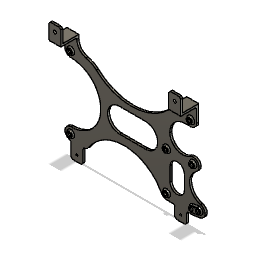
board-mounts (Autodesk Fusion 360 design; units mm, degrees)
Autodesk Fusion 360 part; units mm, degrees
sketch "test-screw-post" plane through (0, 0, 0) normal (0, 1, 0) x (1, 0, 0)
  line L0 (0, 0) -> (10, 0)
  line L1 (10, 0) -> (10, 10)
  line L2 (10, 10) -> (0, 10)
  line L3 (0, 10) -> (0, 0)
  circle A0 centre (5, 5) radius 1.55
  circle A1 centre (5, 5) radius 3.25
  dimension "d1" = 3.1
  dimension "d2" = 6.5
  dimension "d12" = 10
  constraint horizontal L0
  constraint vertical L1
  constraint horizontal L2
  constraint vertical L3
  constraint coincident L0.start L3.end
  constraint concentric A0 A1
  constraint equal L0 L1
  constraint collinear L0.end L2.end A0.centre
  constraint collinear L0.start L1.end A0.centre
  measures "d1" diameter of A0
  measures "d2" diameter of A1
  measures "d12" distance of L0.start L0.end
extrude "test-screw-post base" add sketch "test-screw-post" along normal blind 2.5 contours L0 L1 L2 L3 makes body 1
extrude "test-screw-post post" add sketch "test-screw-post" along normal blind 5 contours A1 bodies 1
fillet "test-screw-post post filet" radius 1.5 1 edges at (1.9699, 2.5, -6.1753) on bodies 1
chamfer "test-screw-post post hole chamfer" distance 0.75 angle 45 1 edges at (3.5549, 5, -5.5605) on bodies 1
sketch "mosfet-mount" plane through (0, 0, 0) normal (0, 0, 1) x (1, 0, 0)
  line L0 (31.2098, -47.0147) -> (36.1264, -47.3213)
  circle A0 centre (31.2098, -38.8279) radius 3.25
  arc A1 (27.187, -6.2985) -> (38.2098, -17.3213) centre (38.2098, -6.2985) ccw
  circle A2 centre (31.2098, -38.8279) radius 1.55
  arc A3 (23.3796, -41.2179) -> (31.2098, -47.0147) centre (31.2098, -38.8279) ccw
  arc A4 (23.3796, -41.2179) -> (1.2098, -24.8051) centre (1.2098, -47.9846) ccw
  line L1 (13.5336, -24.8051) -> (1.2098, -24.8051)
  line L2 (-11.1141, -24.8051) -> (1.2098, -24.8051)
  line L3 (1.2098, -24.8051) -> (1.2098, -17.3051)
  arc A5 (1.2098, -24.8051) -> (-20.9601, -41.2179) centre (1.2098, -47.9846) ccw
  circle A6 centre (-28.7902, -38.8279) radius 3.25
  circle A7 centre (-28.7902, -38.8279) radius 1.55
  line L4 (-35.7902, -47.0147) -> (-35.7902, -32.0147)
  arc A8 (19.687, 0.7275) -> (1.2098, 19.2047) centre (1.2098, 0.7275) ccw
  line L5 (27.187, 7.8914) -> (27.187, 0.7275)
  arc A9 (38.2098, 18.9143) -> (27.187, 7.8914) centre (38.2098, 7.8914) ccw
  arc A10 (1.2098, 26.7047) -> (23.3796, 43.1174) centre (1.2098, 49.8842) ccw
  line L6 (1.2098, 26.7047) -> (1.2098, 19.2047)
  arc A11 (1.2098, 19.2047) -> (-17.2674, 0.7275) centre (1.2098, 0.7275) ccw
  arc A12 (-20.9601, 43.1174) -> (1.2098, 26.7047) centre (1.2098, 49.8842) ccw
  line L7 (-11.1141, 26.7047) -> (1.2098, 26.7047)
  circle A13 centre (-28.7902, 40.7275) radius 3.25
  circle A14 centre (-28.7902, 40.7275) radius 1.55
  line L8 (-35.7902, 48.9143) -> (-35.7902, 33.9143)
  line L9 (-28.7902, 48.9143) -> (-35.7902, 48.9143)
  arc A15 (-20.9601, 43.1174) -> (-28.7902, 48.9143) centre (-28.7902, 40.7275) ccw
  circle A16 centre (31.2098, 40.7275) radius 3.25
  circle A17 centre (31.2098, 40.7275) radius 1.55
  line L10 (31.2098, 48.9143) -> (40.7098, 48.9143)
  line L11 (38.2098, 48.9143) -> (38.2098, 18.9143)
  line L12 (40.7098, 48.9143) -> (40.7098, 18.9143)
  arc A18 (31.2098, 48.9143) -> (23.3796, 43.1174) centre (31.2098, 40.7275) ccw
  arc A19 (-24.7674, 22.7238) -> (-35.7902, 33.9143) centre (-35.9591, 22.7238) ccw
  arc A20 (-35.7902, -32.0147) -> (-24.7674, -20.8242) centre (-35.9591, -20.8242) ccw
  arc A21 (-17.2674, 1.1721) -> (1.2098, -17.3051) centre (1.2098, 1.1721) ccw
  line L13 (27.187, -6.2985) -> (27.187, 1.1721)
  arc A22 (-28.7902, -47.0147) -> (-20.9601, -41.2179) centre (-28.7902, -38.8279) ccw
  line L14 (-28.7902, -47.0147) -> (-35.7902, -47.0147)
  line L15 (-8.7902, 0.9498) -> (10.2098, 0.9498)
  line L16 (11.2098, 0.9498) -> (-7.7902, 0.9498)
  line L17 (1.2098, 7) -> (1.2098, -7.7588)
  line L18 (-24.7674, 22.7238) -> (-24.7674, 0.7275)
  arc A23 (1.2098, -17.3051) -> (19.687, 1.1721) centre (1.2098, 1.1721) ccw
  line L19 (27.187, 1.1721) -> (19.687, 1.1721)
  line L20 (27.187, 0.7275) -> (19.687, 0.7275)
  line L21 (-24.7674, 1.1721) -> (-17.2674, 1.1721)
  line L22 (-24.7674, 0.7275) -> (-17.2674, 0.7275)
  line L23 (-24.7674, -20.8242) -> (-24.7674, 1.1721)
  line L24 (40.4687, -47.3213) -> (36.1264, -47.3213)
  line L25 (38.2098, -17.3213) -> (38.2098, -47.3213)
  line L26 (40.4687, -17.3213) -> (40.4687, -47.3213)
  line L27 (-35.7902, 48.9143) -> (-43.7902, 48.9143)
  line L28 (-45.7902, 46.9143) -> (-45.7902, 35.9143)
  line L29 (-43.7902, 33.9143) -> (-35.7902, 33.9143)
  line L30 (-35.7902, 33.9143) -> (-35.7902, 48.9143)
  line L31 (-35.7902, -32.0147) -> (-43.7902, -32.0147)
  line L32 (-45.7902, -34.0147) -> (-45.7902, -45.0147)
  line L33 (-43.7902, -47.0147) -> (-35.7902, -47.0147)
  line L34 (-35.7902, -47.0147) -> (-35.7902, -32.0147)
  circle A24 centre (-40.7902, 40.7275) radius 1.25
  circle A25 centre (-40.7902, -38.8279) radius 1.25
  line L35 (-45.7902, 46.9143) -> (-43.7902, 48.9143)
  line L36 (-45.7902, 35.9143) -> (-43.7902, 33.9143)
  line L37 (-45.7902, -34.0147) -> (-43.7902, -32.0147)
  line L38 (-45.7902, -45.0147) -> (-43.7902, -47.0147)
  line L39 (38.2098, 18.9143) -> (40.7098, 18.9143)
  line L40 (38.2098, -17.3213) -> (40.4687, -17.3213)
  point P0 (1.2098, 0.7275)
  point P1 (1.2098, 0.7275)
  dimension "d19" = 3.1
  dimension "d20" = 6.5
  dimension "d11" = 40
  dimension "d23" = 15
  dimension "d24" = 7.5
  dimension "d26" = 8.1868
  dimension "d38" = 30
  dimension "d47" = 2.5
  dimension "d48" = 7
  dimension "d52" = 2.5
  dimension "d53" = 2
  dimension "d54" = 2
  dimension "d56" = 10
  dimension "d57" = 2
  dimension "d58" = 5
  dimension "d59" = 2
  dimension "d60" = 2
  dimension "d136" = 30
  dimension "d137" = 30
  constraint concentric A14 A15
  constraint coincident A13.centre A14.centre
  constraint tangent A15 A19
  constraint tangent A12 A15
  constraint vertical L18
  constraint horizontal L7
  constraint tangent A12 L7
  constraint tangent A19 L18
  constraint coincident P1 P0
  constraint horizontal L9
  constraint vertical L9.start A13.centre
  constraint coincident A10.start L7
  constraint perpendicular L6 L7
  constraint horizontal L22
  constraint horizontal P1 L18.end
  constraint coincident A10.start L6.start
  constraint coincident A11.end L22.end
  constraint coincident L8.start L9
  constraint coincident L8.end A19
  constraint perpendicular L8 L9
  constraint horizontal L15
  constraint vertical P1 A10.start
  constraint equal L6 L22
  constraint symmetric A7 A14 L15
  constraint symmetric A6 A13 L15
  constraint symmetric A19.start A20.end L15
  constraint symmetric L8.end L4.end L15
  constraint symmetric A19 A20 L15
  constraint symmetric A12.start A5.end L15
  constraint symmetric A4.end A10.start L15
  constraint symmetric A5 A12 L15
  constraint symmetric L21.start L18.end L15
  constraint symmetric L7.start L2.start L15
  constraint symmetric L9.start A22.start L15
  constraint symmetric L8.start L4.start L15
  constraint symmetric A15 A22 L15
  constraint symmetric A10.start A4.end L15
  constraint symmetric A8.end L3.end L15
  constraint symmetric A11.end A21.start L15
  constraint symmetric A11 A21 L15
  constraint symmetric L4.start L8.start L15
  constraint perpendicular L15 L17
  constraint vertical A21.centre L17.start
  constraint symmetric A14 A17 L17
  constraint symmetric A13 A16 L17
  constraint symmetric A12.start A10.end L17
  constraint symmetric A10.start L6.start L17
  constraint symmetric A10 A12 L17
  constraint symmetric L18.end L5.end L17
  constraint symmetric L9.start L10.start L17
  constraint symmetric A15 A18 L17
  constraint symmetric A8.end L6.end L17
  constraint symmetric A11.end A8.start L17
  constraint symmetric A8.start A11.end L17
  constraint symmetric A8 A11 L17
  constraint symmetric L11.start L8.start L17
  constraint symmetric L15.start L16.start L17
  constraint symmetric L15.end L16.end L17
  constraint symmetric L1.start L2.start L17
  constraint symmetric L3.end A21.end L17
  constraint symmetric A23.end A21.start L17
  constraint symmetric A0 A6 L17
  constraint symmetric A2 A7 L17
  constraint symmetric A5.end A3.start L17
  constraint symmetric A4.end L1.end L17
  constraint symmetric A4 A5 L17
  constraint symmetric A22.start L0.start L17
  constraint symmetric A21 L17 A23
  constraint symmetric L21.start L13.end L17
  constraint symmetric A3 A22 L17
  constraint coincident L8.start L9.end
  constraint coincident L8.end A19.end
  constraint coincident L0.end L24.end
  constraint horizontal L24
  constraint coincident L24 L25.end
  constraint perpendicular L24 L25
  constraint perpendicular L24 L26
  constraint horizontal L27
  constraint vertical L28
  constraint horizontal L29
  constraint vertical L30
  constraint horizontal L31
  constraint vertical L32
  constraint horizontal L33
  constraint vertical L34
  constraint coincident L4.start L14.end
  constraint equal A24 A25
  constraint vertical L27.end L29.start
  constraint horizontal A13.centre A24.centre
  constraint vertical A24.centre A25.centre
  constraint vertical L31.end L33.start
  constraint vertical L29.start L31.end
  constraint vertical L28.end L32.start
  constraint horizontal A6.centre A25.centre
  constraint coincident L11.start L10
  constraint coincident L10.end L12.start
  constraint vertical L12
  constraint coincident A9.start L11.end
  constraint vertical L5
  constraint tangent L5 A9
  constraint tangent A9 L39
  constraint horizontal L39
  constraint horizontal L40
  constraint tangent A1 L13
  constraint horizontal A1.end L25.start
  constraint vertical L13
  constraint coincident A1.end L25.start
  constraint vertical L11
  constraint vertical A9.start A1.end
  constraint tangent A1 L40
  measures "d19" diameter of A14
  measures "d20" diameter of A13
  measures "d11" vertical distance of A13.centre P1
  measures "d23" distance of L8.end L8.start
  measures "d24" distance of A10.start A8.end
  measures "d26" radius of A15
  measures "d38" horizontal distance of A13.centre P1
  measures "d47" distance of L10.end L11.start
  measures "d48" horizontal distance of A13.centre L8.start
  measures "d52" diameter of A24
  measures "d53" vertical distance of L28.start L27.end
  measures "d54" vertical distance of L28.end L29.start
  measures "d56" horizontal distance of L8.start L28.start
  measures "d57" horizontal distance of L28.end L29.start
  measures "d58" horizontal distance of A24.centre L28.start
  measures "d59" vertical distance of L32.start L31.end
  measures "d60" vertical distance of L32.end L33.start
  measures "d136" distance of L24.start L26.start
  measures "d137" distance of L10.end L12.end
extrude "mosfet-mount (1)" add sketch "mosfet-mount" along normal blind 2.5 separate body contours L0 A1 A3 A4 L3 A8 L13 A23 L20 L24 L25 | L3 A5 L4 A11 A20 A21 A22 L14 L22 L23 L34 | L6 A11 A12 L8 L9 A15 A19 A21 L18 L21 L30 | A11 A21 L18 L21 L22 L23 | A8 L5 L13 A23 L19 L20 | A8 L5 A9 A10 L6 L10 L11 A18 A23 L19 | L4 L31 L32 L33 L34 L37 L38 | L8 L27 L28 L29 L30 L35 L36 makes body 2
extrude "mosfet-mount post" add sketch "mosfet-mount" along normal blind 5 contours A0 | A6 | A13 | A16 bodies 2
fillet "mosfet-mount post filet" radius 1.5 4 edges at (-31.8203, -37.6527, 2.5) (-31.8203, 41.9027, 2.5) (28.1797, 41.9027, 2.5) (28.1797, -37.6527, 2.5) on bodies 2
chamfer "mosfet-mount post hole chamfer" distance 0.75 angle 45 4 edges at (29.7647, 41.288, 5) (-30.2353, 41.288, 5) (-30.2353, -38.2674, 5) (29.7647, -38.2674, 5) on bodies 2
extrude "mosfet-mount 2020 attachment tabs" add sketch "mosfet-mount" along normal blind 20 contours L24 L25 L26 L40 | L10 L11 L12 L39 bodies 2
sketch "mosfet-mount 2020 screw hole" plane through (38.2098, 0, 0) normal (-1, 0, 0) x (0, 0, 1)
  line L0 (2.5, 48.9143) -> (2.5, 18.9143)
  line L1 (20, 18.9143) -> (20, 48.9143)
  line L2 (20, 48.9143) -> (2.5, 48.9143)
  circle A0 centre (10, 28.9143) radius 1.875
  circle A1 centre (10, -27.3213) radius 1.875
  line L3 (2.5, 18.9143) -> (20, 18.9143)
  line L4 (2.5, 48.9143) -> (2.5, 18.9143)
  line L5 (2.5, 18.9143) -> (20, 18.9143)
  line L6 (20, 18.9143) -> (20, 48.9143)
  line L7 (20, 48.9143) -> (2.5, 48.9143)
  point P0 (0, 33.914)
  point P1 (0, -47.0147)
  point P2 (20, -47.3213)
  point P3 (20, -17.3213)
  dimension "d43" = 3.75
  dimension "d44" = 10
  dimension "d138" = 10
  dimension "d139" = 10
  constraint equal A0 A1
  constraint vertical A0.centre A1.centre
  measures "d43" diameter of A0
  measures "d44" horizontal distance of L1.end A0.centre
  measures "d138" vertical distance of L1.start A0.centre
  measures "d139" vertical distance of A1.centre P3
extrude "Extrude6" cut sketch "mosfet-mount 2020 screw hole" against normal through all contours A0 | A1 bodies 2
fillet "mosfet-mount tab filet" radius 2 2 edges at (38.2098, -32.3213, 2.5) (38.2098, 33.9143, 2.5) on bodies 2
chamfer "Chamfer6" distance 15 angle 45 2 edges at (39.3392, -47.3213, 20) (39.4598, 48.9143, 20) on bodies 2
chamfer "mosfet-mount minor chamfer" distance 2 angle 45 2 edges at (39.3392, -17.3213, 20) (39.4598, 18.9143, 20) on bodies 2
sketch "mb8-mount" plane through (0, 0, 0) normal (0, 0, 1) x (1, 0, 0)
  line L0 (18.0353, -18.811) -> (7.0353, -18.811)
  line L1 (20.0353, -16.811) -> (18.0353, -18.811)
  line L2 (98.6501, 68.0356) -> (66, 68.0356)
  line L3 (162.5, 134) -> (160.5, 136)
  arc A0 (66, 68.0356) -> (66, 37.9644) centre (66, 53) ccw
  arc A1 (157.94, -3.81) -> (159.2205, -3.6999) centre (157.94, 3.69) ccw
  circle A2 centre (12.5353, -11.311) radius 1.25
  line L4 (149.5, 136) -> (147.5, 134)
  arc A3 (135.0353, -5.81) -> (133.0353, -3.81) centre (133.0353, -5.81) ccw
  arc A4 (166.0549, 1.7977) -> (164.9451, 8.2023) centre (165.5, 5) ccw
  arc A5 (129, 17.4847) -> (147.05, 17.4847) centre (138.025, 17.4847) ccw
  line L5 (150.0353, -5.81) -> (150.0353, -16.811)
  line L6 (166.0549, 1.7977) -> (158.4949, 0.4877)
  arc A6 (128.7928, 70.7811) -> (153.7221, 57.8916) centre (144.7477, 71.0868) ccw
  circle A7 centre (157.94, 51.69) radius 3.25
  arc A8 (155, 90.5) -> (162.5, 98) centre (155, 98) ccw
  line L7 (149.5, 136) -> (160.5, 136)
  arc A9 (161.9954, 45.381) -> (167.3573, 12.2664) centre (171.888, 29.9914) ccw
  line L8 (150.0353, -16.811) -> (148.0353, -18.811)
  line L9 (148.0353, -18.811) -> (137.0353, -18.811)
  circle A10 centre (142.5353, -11.311) radius 1.25
  line L10 (12.5, 118) -> (-2.5, 118)
  arc A11 (21.7902, 0.5723) -> (27.5631, 4.2202) centre (20.8091, 8.5168) ccw
  line L11 (7.0353, -18.811) -> (5.0353, -16.811)
  line L12 (12.5, 134) -> (10.5, 136)
  line L13 (-2.5, 98) -> (-2.5, 118)
  line L14 (129, 35) -> (129, 17.4847)
  circle A12 centre (124.94, 3.69) radius 1.55
  circle A13 centre (124.94, 51.69) radius 3.25
  arc A14 (5, 15.5) -> (5, 90.5) centre (5, 53) ccw
  arc A15 (5.0353, -0.6626) -> (3.9611, 0.5723) centre (3.7884, -0.6626) ccw
  circle A16 centre (155, 98) radius 3.25
  line L15 (152.0353, -3.81) -> (157.94, -3.81)
  line L16 (138.025, 35) -> (138.025, 17.4847) construction
  arc A17 (36.7596, 92.8575) -> (24.0633, 99.4776) centre (18.2949, 72.9301) ccw
  circle A18 centre (5, 98) radius 3.25
  circle A19 centre (5, 98) radius 1.55
  circle A20 centre (5, 8) radius 1.55
  line L17 (66, 37.9644) -> (98.6501, 37.9644)
  arc A21 (-2.5, 98) -> (5, 90.5) centre (5, 98) ccw
  line L18 (137.0353, -18.811) -> (135.0353, -16.811)
  arc A22 (21.7902, 0.5723) -> (20.0353, -1.4126) centre (22.0353, -1.4126) ccw
  line L19 (-0.5, 136) -> (10.5, 136)
  line L20 (12.5, 134) -> (12.5, 118)
  circle A23 centre (165.5, 5) radius 1.55
  line L21 (147.05, 17.4847) -> (147.05, 35)
  line L22 (162.5, 118) -> (147.5, 118)
  arc A24 (161.9954, 45.381) -> (153.7221, 57.8916) centre (157.94, 51.69) ccw
  arc A25 (136.7325, 99.674) -> (125.3321, 93.2519) centre (143.9735, 73.4898) ccw
  arc A26 (152.0353, -3.81) -> (150.0353, -5.81) centre (152.0353, -5.81) ccw
  line L23 (124.94, -3.81) -> (133.0353, -3.81)
  arc A27 (98.6501, 37.9644) -> (98.6501, 68.0356) centre (98.6501, 53) ccw
  arc A28 (148.1374, 90.5) -> (128.7928, 70.7811) centre (148.1374, 71.1518) ccw
  circle A29 centre (155, 128) radius 1.875
  circle A30 centre (157.94, 3.69) radius 1.55
  circle A31 centre (124.94, 51.69) radius 1.55
  line L24 (155, 90.5) -> (153.7366, 90.5)
  circle A32 centre (155, 98) radius 1.55
  line L25 (147.5, 113.8232) -> (147.5, 118)
  circle A33 centre (157.94, 51.69) radius 1.55
  circle A34 centre (124.94, 3.69) radius 3.25
  line L26 (135.0353, -16.811) -> (135.0353, -5.81)
  arc A35 (166.7805, -2.3899) -> (167.3573, 12.2664) centre (165.5, 5) ccw
  arc A36 (147.05, 35) -> (129, 35) centre (138.025, 35) ccw
  line L27 (153.7366, 90.5) -> (148.1374, 90.5)
  arc A37 (157.3851, 6.8923) -> (158.4949, 0.4877) centre (157.94, 3.69) ccw
  arc A38 (136.7325, 99.674) -> (147.5, 113.8232) centre (132.8197, 113.8232) ccw
  line L28 (157.3851, 6.8923) -> (164.9451, 8.2023)
  line L29 (162.5, 134) -> (162.5, 118)
  line L30 (162.5, 115.5) -> (147.5, 115.5)
  line L31 (147.5, 118) -> (147.5, 134)
  line L32 (162.5, 118) -> (147.5, 118)
  line L33 (162.5, 98) -> (162.5, 118)
  arc A39 (118.2833, 0.2348) -> (124.94, -3.81) centre (124.94, 3.69) ccw
  line L34 (159.2205, -3.6999) -> (166.7805, -2.3899)
  line L35 (-0.5, 136) -> (-2.5, 134)
  arc A40 (118.2833, 0.2348) -> (27.5631, 4.2202) centre (71.7752, -23.9055) ccw
  line L36 (20.0353, -16.811) -> (20.0353, -1.4126)
  line L37 (98.6501, 53) -> (66, 53) construction
  line L38 (-2.5, 118) -> (-2.5, 134)
  line L39 (12.5, 118) -> (-2.5, 118)
  line L40 (12.5, 118) -> (12.5, 113.8232)
  line L41 (12.5, 115.5) -> (-2.5, 115.5)
  circle A41 centre (5, 8) radius 3.25
  arc A42 (12.5, 113.8232) -> (24.0633, 99.4776) centre (27.1803, 113.8232) ccw
  arc A43 (5, 15.5) -> (3.9611, 0.5723) centre (5, 8) ccw
  circle A44 centre (5, 128) radius 1.875
  arc A45 (36.7596, 92.8575) -> (125.3321, 93.2519) centre (80.8349, 140.4243) ccw
  line L42 (5.0353, -16.811) -> (5.0353, -0.6626)
  point P0 (138.025, 26.2424)
  point P1 (82.325, 53)
  dimension "d65" = 8
  dimension "d66" = 5
  dimension "d67" = 98
  dimension "d68" = 165.5
  dimension "d69" = 5
  dimension "d70" = 155
  dimension "d71" = 3.1
  dimension "d72" = 3.1
  dimension "d13" = 3.69
  dimension "d14" = 51.69
  dimension "d15" = 124.94
  dimension "d16" = 157.94
  dimension "d17" = 6.5
  dimension "d18" = 15
  dimension "d79" = 6.5
  dimension "d80" = 7.5
  dimension "d25" = 7.56
  dimension "d27" = 7.5
  dimension "d83" = 7.5
  dimension "d84" = 7.5
  dimension "d85" = 20
  dimension "d86" = 2.5
  dimension "d87" = 7.5
  dimension "d88" = 7.5
  dimension "d89" = 7.5
  dimension "d90" = 10
  dimension "d91" = 10
  dimension "d49" = 7.5
  dimension "d50" = 3.75
  dimension "d94" = 2
  dimension "d55" = 2
  dimension "d96" = 2
  dimension "d97" = 18
  dimension "d98" = 18
  dimension "d99" = 2
  dimension "d100" = 2
  dimension "d61" = 2
  dimension "d62" = 2
  dimension "d103" = 2.5
  dimension "d104" = 2.5
  dimension "d105" = 2
  dimension "d73" = 2
  dimension "d74" = 2
  dimension "d75" = 2
  dimension "d77" = 7.5
  dimension "d78" = 7.5
  dimension "d111" = 2
  dimension "d112" = 2
  dimension "d81" = 2
  dimension "d82" = 15
  dimension "d115" = 7.5
  dimension "d116" = 7.5
  dimension "d117" = 2
  dimension "d118" = 15
  dimension "d119" = 130
  dimension "d120" = 2
  constraint vertical A18.centre A20.centre
  constraint horizontal A8.centre A18.centre
  constraint equal A19 A20
  constraint equal A19 A32
  constraint equal A23 A32
  constraint horizontal A13.centre A7.centre
  constraint vertical A13.centre A12.centre
  constraint horizontal A1.centre A12.centre
  constraint equal A31 A33
  constraint equal A30 A33
  constraint equal A12 A30
  constraint vertical A1.centre A7.centre
  constraint concentric A20 A41
  constraint concentric A20 A43
  constraint concentric A18 A19
  constraint concentric A18 A21
  constraint concentric A16 A32
  constraint concentric A8 A32
  constraint concentric A4 A23
  constraint concentric A30 A37
  constraint concentric A12 A34
  constraint concentric A7 A33
  constraint concentric A7 A24
  constraint concentric A13 A31
  constraint equal A18 A41
  constraint equal A16 A18
  constraint equal A4 A16
  constraint equal A7 A13
  constraint equal A7 A34
  constraint equal A34 A37
  constraint equal A21 A43
  constraint equal A8 A24
  constraint concentric A1 A37
  constraint tangent A1 L34
  constraint coincident A4.centre A23.centre
  constraint vertical A14.end A18.centre
  constraint vertical A14.centre A14.end
  constraint vertical A14.centre A14.start
  constraint tangent A1 L23
  constraint tangent A17 A45
  constraint tangent A25 A45
  constraint vertical A8.start A8.centre
  constraint coincident A12.centre A34.centre
  constraint coincident L23.start A39.end
  constraint coincident A39.start A40.start
  constraint tangent A39 A40
  constraint tangent L2 A0
  constraint tangent A0 L17
  constraint parallel L2 L17
  constraint tangent L17 A27
  constraint tangent L2 A27
  constraint horizontal L37
  constraint midpoint P1 L37
  constraint horizontal A14.centre P1
  constraint tangent A8 L24
  constraint parallel L24 L27
  constraint tangent A6 A24
  constraint tangent A28 L27
  constraint coincident A6.start A28.end
  constraint tangent A6 A28
  constraint tangent A9 A24
  constraint tangent A5 L14
  constraint tangent A5 L21
  constraint parallel L14 L21
  constraint tangent L21 A36
  constraint tangent L14 A36
  constraint vertical L16
  constraint midpoint P0 L16
  constraint tangent A4 L28
  constraint tangent L6 A37
  constraint tangent A4 L6
  constraint tangent A37 L28
  constraint coincident A9.end A35.end
  constraint tangent A9 A35
  constraint horizontal L22
  constraint tangent A8 L33
  constraint coincident L22.start L29.end
  constraint tangent L13 A21
  constraint perpendicular L13 L22
  constraint coincident L10.end L13.end
  constraint coincident L30.start L33
  constraint coincident L41.end L13
  constraint perpendicular L13 L30
  constraint perpendicular L22 L25
  constraint coincident A38.end L25
  constraint coincident L25.start A38
  constraint tangent L25 A38
  constraint tangent A25 A38
  constraint coincident L10.start L22
  constraint coincident L30.end L25
  constraint coincident L41.start L40
  constraint collinear L30 L41
  constraint collinear L10 L22
  constraint coincident A17.end A42.end
  constraint vertical L40
  constraint tangent L40 A42
  constraint tangent A17 A42
  constraint horizontal L40.end L25.start
  constraint equal A38 A42
  constraint equal A17 A25
  constraint horizontal L32
  constraint vertical L31
  constraint horizontal L7
  constraint vertical L29
  constraint horizontal L39
  constraint vertical L38
  constraint horizontal L19
  constraint vertical L20
  constraint equal A29 A44
  constraint vertical L33
  constraint perpendicular L3 L4
  constraint coincident L22.end L25.end
  constraint horizontal L23
  constraint perpendicular L5 L23
  constraint perpendicular L5 L9
  constraint perpendicular L23 L26
  constraint horizontal L0
  constraint vertical L42
  constraint perpendicular L0 L36
  constraint collinear L15 L23
  constraint perpendicular L1 L11
  constraint horizontal L9.end L0.start
  constraint coincident L15.start A26
  constraint coincident L15.start A26.start
  constraint tangent L5 A26
  constraint tangent L15 A26
  constraint coincident A3.end L23
  constraint coincident L23.end A3
  constraint tangent A3 L23
  constraint tangent A3 L26
  constraint equal A3 A26
  constraint tangent A11 A22
  constraint tangent A22 L36
  constraint coincident L42.end A15
  constraint tangent A15 A43
  constraint tangent A15 L42
  constraint coincident A15.start L42.end
  constraint horizontal A15.end A11.start
  constraint tangent A11 A40
  measures "d65" vertical distance of origin A20.centre
  measures "d66" horizontal distance of origin A20.centre
  measures "d67" vertical distance of origin A18.centre
  measures "d68" horizontal distance of origin A4.centre
  measures "d69" vertical distance of origin A4.centre
  measures "d70" horizontal distance of origin A8.centre
  measures "d71" diameter of A20
  measures "d72" diameter of A31
  measures "d13" vertical distance of origin A12.centre
  measures "d14" vertical distance of origin A13.centre
  measures "d15" horizontal distance of origin A12.centre
  measures "d16" horizontal distance of origin A1.centre
  measures "d17" diameter of A41
  measures "d18" diameter of A43
  measures "d79" diameter of A13
  measures "d80" radius of A35
  measures "d25" horizontal distance of A1.end A35.start
  measures "d27" radius of A1
  measures "d83" radius of A39
  measures "d84" radius of A8
  measures "d85" vertical distance of A8.centre L22.start
  measures "d86" distance of L22.start L30.start
  measures "d87" horizontal distance of A8.centre L25.start
  measures "d88" horizontal distance of A18.centre L41.start
  measures "d89" horizontal distance of L22.start A29.centre
  measures "d90" vertical distance of L22.start A29.centre
  measures "d91" vertical distance of A44.centre L10.start
  measures "d49" horizontal distance of A44.centre L10.start
  measures "d50" diameter of A44
  measures "d94" horizontal distance of L3.end L3.start
  measures "d55" horizontal distance of L4.start L4.end
  measures "d96" vertical distance of L3.end L3.start
  measures "d97" vertical distance of L22.start L3.end
  measures "d98" vertical distance of L10.end L19.start
  measures "d99" vertical distance of L12.end L12.start
  measures "d100" horizontal distance of L12.end L12.start
  measures "d61" horizontal distance of L35.end L19.start
  measures "d62" vertical distance of L35.end L19.start
  measures "d103" diameter of A10
  measures "d104" diameter of A2
  measures "d105" vertical distance of L5.end L8.end
  measures "d73" horizontal distance of L5.end L8.end
  measures "d74" horizontal distance of L9.end L18.end
  measures "d75" vertical distance of L9.end L18.end
  measures "d77" vertical distance of A10.centre L8.end
  measures "d78" horizontal distance of A10.centre L5.end
  measures "d111" horizontal distance of L0.start L1.start
  measures "d112" horizontal distance of L0.end L11.end
  measures "d81" vertical distance of L0.end L11.end
  measures "d82" distance of L11.end L1.start
  measures "d115" horizontal distance of L1.start A2.centre
  measures "d116" vertical distance of L0.start A2.centre
  measures "d117" radius of A26
  measures "d118" distance of L18.end L5.end
  measures "d119" distance of A10.centre A2.centre
  measures "d120" radius of A22
extrude "mb8-mount base" add sketch "mb8-mount" along normal blind 2.5 separate body contours L0 L1 A1 A3 L5 A6 A8 A9 L8 L9 A11 L11 L13 A14 A15 L15 A17 A21 L18 A22 A24 A25 A26 L23 A28 L24 L25 L26 A35 L27 A38 L30 L33 A39 L34 A40 L36 L40 L41 A42 A43 A45 L42 makes body 3
extrude "mb8-mount posts" add sketch "mb8-mount" along normal blind 5 contours A4 L6 A37 L28 | A7 | A13 | A16 | A18 | A34 | A41 bodies 3
fillet "mb8-mount post filet" radius 1.5 10 edges at (1.9699, 9.1753, 2.5) (1.9699, 99.1753, 2.5) (151.9699, 99.1753, 2.5) (154.9099, 52.8653, 2.5) (121.9099, 52.8653, 2.5) (121.9099, 4.8653, 2.5) (168.7023, 5.5549, 2.5) (162.2749, 1.1427, 2.5) (154.7377, 3.1351, 2.5) (161.1651, 7.5473, 2.5) on bodies 3
chamfer "mb8-mount post hole chamfer" distance 0.75 angle 45 8 edges at (3.5549, 8.5605, 5) (3.5549, 98.5605, 5) (153.5549, 98.5605, 5) (123.4949, 52.2505, 5) (156.4949, 52.2505, 5) (123.4949, 4.2505, 5) (164.0549, 5.5605, 5) (156.4949, 4.2505, 5) on bodies 3
extrude "mb8-mount tab vertical" add sketch "mb8-mount" along normal blind 20 contours L10 L13 L39 L40 L41 | L22 L25 L30 L32 L33 bodies 3
extrude "mb8-mount tab" add sketch "mb8-mount" along normal blind 2.5 from surface at 20 contours L10 L13 L39 L40 L41 | L10 L12 L19 L20 L35 L38 L39 | L22 L25 L30 L32 L33 | L3 L4 L7 L22 L29 L31 L32 bodies 3
fillet "mb8-mount tab filet" radius 2 2 edges at (5, 115.5, 2.5) (155, 115.5, 2.5) on bodies 3
hidden bodies 1 2
equation "d1 = postHoleD"
equation "d2 = postD"
equation "d3 = baseH"
equation "d5 = postH"
equation "d8 = postFilet"
equation "d10 = postHoleChamfer"
equation "baseW = 10 mm"
equation "d12 = baseW"
equation "postD = 6.5 mm"
equation "postFilet = 1.5 mm"
equation "postH = 5 mm"
equation "postHoleD = 3.1 mm"
equation "postHoleChamfer = 0.75 mm"
equation "baseH = 2.5 mm"
equation "d19 = postHoleD"
equation "d20 = postD"
equation "d31 = baseH"
equation "d33 = postH"
equation "d36 = postFilet"
equation "d39 = postHoleChamfer"
equation "screwD2020 = 3.75 mm"
equation "d43 = screwD2020"
equation "screwAttachment = 2.5 mm"
equation "d52 = screwAttachment"
equation "d71 = postHoleD"
equation "d72 = postHoleD"
equation "d17 = postD"
equation "d79 = postD"
equation "d50 = screwD2020"
equation "d103 = screwAttachment"
equation "d104 = screwAttachment"
equation "d121 = baseH"
equation "d123 = postH"
equation "d126 = postFilet"
equation "d127 = postHoleChamfer"
equation "d131 = baseH"
named bodies: "test-screw-post", "mosfet-mount", "mb8-mount"
